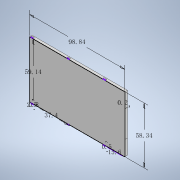
# Autodesk Inventor part: screen
Saved by Autodesk Inventor 2022 (Build 260153000, 153)
## iProperties
Created: 2022-06-18
Part Number: screen
Material: 常规
Document SubType Name: Modeling
Designer: yangmc
Density: 1 g/cm^3
Appearance: 默认
Author: yangmc
Autodesk Inventor part; units mm, degrees
ref_plane "YZ Plane" through (0, 0, 0) normal (1, 0, 0) x (0, 1, 0)
ref_plane "XZ Plane" through (0, 0, 0) normal (0, 1, 0) x (-1, 0, 0)
ref_plane "XY Plane" through (0, 0, 0) normal (0, 0, 1) x (1, 0, 0)
sketch "草图1" plane through (0, 0, 0) normal (0, 0, 1) x (1, 0, 0)
  line L0 (0, 0) -> (98.84, 0)
  line L1 (98.84, 0) -> (98.84, 58.34)
  line L2 (98.84, 58.34) -> (0, 58.34)
  line L3 (0, 58.34) -> (0, 0)
  line L4 (1.44, 0) -> (3.94, 0)
  line L5 (3.94, 0) -> (3.94, -0.8)
  line L6 (3.94, -0.8) -> (1.44, -0.8)
  line L7 (1.44, -0.8) -> (1.44, 0)
  line L8 (41.34, -0.8) -> (38.84, -0.8)
  line L9 (38.84, 0) -> (41.34, 0)
  line L10 (41.34, 0) -> (41.34, -0.8)
  line L11 (38.84, -0.8) -> (38.84, 0)
  line L12 (78.74, -0.8) -> (76.24, -0.8)
  line L13 (76.24, 0) -> (78.74, 0)
  line L14 (78.74, 0) -> (78.74, -0.8)
  line L15 (76.24, -0.8) -> (76.24, 0)
  line L16 (3.94, 58.34) -> (1.44, 58.34)
  line L17 (1.44, 59.14) -> (3.94, 59.14)
  line L18 (3.94, 59.14) -> (3.94, 58.34)
  line L19 (1.44, 58.34) -> (1.44, 59.14)
  line L20 (41.34, 58.34) -> (38.84, 58.34)
  line L21 (38.84, 59.14) -> (41.34, 59.14)
  line L22 (41.34, 59.14) -> (41.34, 58.34)
  line L23 (38.84, 58.34) -> (38.84, 59.14)
  line L24 (78.74, 58.34) -> (76.24, 58.34)
  line L25 (76.24, 59.14) -> (78.74, 59.14)
  line L26 (78.74, 59.14) -> (78.74, 58.34)
  line L27 (76.24, 58.34) -> (76.24, 59.14)
  line L28 (96.16, 0) -> (80.56, 0)
  line L29 (80.56, 0) -> (80.56, -0.5)
  line L30 (80.56, -0.5) -> (96.16, -0.5)
  line L31 (96.16, -0.5) -> (96.16, 0)
  line L32 (98.84, 15.5477) -> (99.04, 15.5477)
  line L33 (99.04, 15.5477) -> (99.04, 43.1523)
  line L34 (99.04, 43.1523) -> (98.84, 43.1523)
  line L35 (98.84, 43.1523) -> (98.84, 15.5477)
  point P0 (1.44, 58.34)
  dimension "d0" = 98.84
  dimension "d1" = 58.34
  dimension "d2" = 2.5
  dimension "d3" = 0.8
  dimension "d6" = 37.4
  dimension "d9" = 59.14
  dimension "d12" = 15.6
  dimension "d13" = 0.5
  dimension "d27" = 0.2
  constraints: 72 end point, 8 parallel, 5 horizontal, 4 perpendicular, 2 collinear, 1 point on line, 1 vertical, 38 other
  measures "d0" distance of L2.end L1.end
  measures "d1" distance of L1.end L0.end
  measures "d2" distance of L5.end L6.end
  measures "d3" distance of L4.end L5.end
  measures "d6" distance of L5.end L8.start
  measures "d9" distance of L5.end L16.start
  measures "d12" distance of L30.end L29.end
  measures "d13" distance of L29.end L28.end
  measures "d27" distance of L34.end L33.end
extrude "拉伸1" add sketch "草图1" against normal blind 2.72 contours L3 L2 L1 L0
extrude "拉伸2" add sketch "草图1" against normal blind 0.8 contours L0 L5 L6 L7 | L19 L17 L18 L2 | L0 L10 L8 L11 | L23 L21 L22 L2 | L0 L14 L12 L15 | L27 L25 L26 L2
extrude "拉伸3" add sketch "草图1" against normal blind 0.1 contours L0 L31 L30 L29
split body "分割1" sketch "草图1" result two bodies curves L6 L7 L4 L5 first body at (27.2067, 19.4467, -0.5)
split body "分割2" sketch "草图1" result two bodies bodies 2 curves L11 L9 L10 L8 first body at (27.2067, 19.4467, -0.5)
split body "分割3" sketch "草图1" result two bodies bodies 4 curves L12 L15 L13 L14 first body at (27.2067, 19.4467, -0.5)
split body "分割4" sketch "草图1" result two bodies bodies 6 curves L30 L31 L28 L29 first body at (85.76, -0.1667, -0.02)
split body "分割5" sketch "草图1" result two bodies bodies 9 curves L17 L18 L16 L19 first body at (27.2067, 19.4467, -0.5)
split body "分割6" sketch "草图1" result two bodies bodies 10 curves L21 L22 L20 L23 first body at (27.2067, 19.4467, -0.5)
split body "分割7" sketch "草图1" result two bodies bodies 12 curves L25 L26 L24 L27 first body at (27.2067, 19.4467, -0.5)
move or copy body "移动实体1" bodies to move or copy 3 copy no translate (0, 0, -0.24)
move or copy body "移动实体2" bodies to move or copy 5 copy no translate (0, 0, -0.24)
move or copy body "移动实体3" bodies to move or copy 7 copy no translate (0, 0, -0.24)
move or copy body "移动实体4" bodies to move or copy 8 copy no translate (0, 0, -2.62)
move or copy body "移动实体5" bodies to move or copy 11 copy no translate (0, 0, -0.24)
move or copy body "移动实体6" bodies to move or copy 13 copy no translate (0, 0, -0.24)
move or copy body "移动实体7" bodies to move or copy 15 copy no translate (0, 0, -0.24)
extrude "拉伸4" add sketch "草图1" against normal blind 2.72 contours L34 L33 L32 L1 bodies 14
